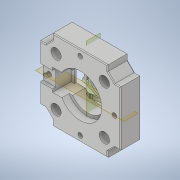
# Autodesk Inventor part: 20_Cube_Insert_VCA_base_upper_v0
Saved by Autodesk Inventor 2022.3 (Build 263350000, 350)
## iProperties
Created: 2019-07-01
Part Number: 20_Cube_Insert_VCA_base_upper_v0
Material: Generic
Document SubType Name: Modeling
Designer: diederichbenedict
Density: 1 g/cm^3
Appearance: Default
Author: diederichbenedict
Autodesk Inventor part; units mm, degrees
ref_plane "YZ Plane" through (0, 0, 0) normal (1, 0, 0) x (0, 1, 0)
ref_plane "XZ Plane" through (0, 0, 0) normal (0, 1, 0) x (-1, 0, 0)
ref_plane "Work Plane1" through (-56.3599, 0, 22) normal (0, 0, -1) x (-1, 0, 0)
sketch "Sketch1" plane through (-56.3599, 0, 22) normal (0, 0, -1) x (-1, 0, 0)
  line L0 (-4.0299, -0.3538) -> (-2.2322, 1.4439) construction
  arc A0 (-1.4439, 2.2322) -> (-2.2322, 1.4439) centre (-0.9299, 0.9299) ccw construction
  line L1 (-1.4439, 2.2322) -> (0.3538, 4.0299) construction
  line L2 (-37.8299, 42.8299) -> (-37.8299, 37.8299) construction
  line L3 (-37.8299, 37.8299) -> (-42.9208, 37.8299) construction
  line L4 (-37.8299, 42.2137) -> (-37.8299, 45.8299) construction
  line L5 (-37.8299, 45.8299) -> (-4.0299, 45.8299) construction
  line L6 (-4.0299, 45.8299) -> (-4.0299, 42.2137) construction
  line L7 (-4.0299, 4.0299) -> (0.3538, 4.0299) projected
  circle A1 centre (-20.9299, 20.9299) radius 17.5 projected
  line L8 (-20.9299, 58.9723) -> (17.1124, 20.9299) construction
  line L9 (17.1124, 20.9299) -> (-20.9299, -17.1124) construction
  line L10 (-20.9299, -17.1124) -> (-58.9723, 20.9299) construction
  line L11 (-58.9723, 20.9299) -> (-20.9299, 58.9723) construction
  line L12 (-20.9299, 58.9723) -> (-20.9299, -17.1124) construction
  line L13 (17.1124, 20.9299) -> (-58.9723, 20.9299) construction
  line L14 (-20.9299, 58.9723) -> (32.8701, 58.9723) construction
  line L15 (-43.4299, 43.4299) -> (1.5701, 43.4299) construction
  line L16 (1.5701, 43.4299) -> (1.5701, -1.5701) construction
  line L17 (1.5701, -1.5701) -> (-43.4299, -1.5701) construction
  line L18 (-43.4299, -1.5701) -> (-43.4299, 43.4299) construction
  line L19 (-43.4299, 43.4299) -> (1.5701, -1.5701) construction
  line L20 (1.5701, 43.4299) -> (-43.4299, -1.5701) construction
  line L21 (-43.4299, 5.3876) -> (-43.4299, 36.4723)
  line L22 (-43.4299, 36.4723) -> (-36.4723, 43.4299)
  line L23 (-36.4723, 43.4299) -> (-5.3876, 43.4299)
  line L24 (-5.3876, 43.4299) -> (1.5701, 36.4723)
  line L25 (1.5701, 36.4723) -> (1.5701, 5.3876)
  line L26 (1.5701, 5.3876) -> (-5.3876, -1.5701)
  line L27 (-5.3876, -1.5701) -> (-36.4723, -1.5701)
  line L28 (-36.4723, -1.5701) -> (-43.4299, 5.3876)
  line L29 (-4.0299, 42.2137) -> (-37.8299, 42.2137) projected
  line L30 (-4.0299, -0.3538) -> (-4.0299, 4.0299) projected
  circle A2 centre (-20.9299, 20.9299) radius 1.5
  line L31 (-10.9299, 10.9299) -> (-30.9299, 10.9299) construction
  line L32 (-30.9299, 10.9299) -> (-30.9299, 30.9299) construction
  line L33 (-30.9299, 30.9299) -> (-10.9299, 30.9299) construction
  line L34 (-10.9299, 30.9299) -> (-10.9299, 10.9299) construction
  line L35 (-10.9299, 10.9299) -> (-30.9299, 30.9299) construction
  line L36 (-30.9299, 10.9299) -> (-10.9299, 30.9299) construction
  circle A3 centre (-30.9299, 30.9299) radius 1.4
  circle A4 centre (-30.9299, 10.9299) radius 1.4
  circle A5 centre (-10.9299, 10.9299) radius 1.4
  line L37 (-45.8299, 37.8299) -> (-42.0723, 37.8299) construction
  line L38 (-42.1723, 37.7299) -> (-45.8299, 37.7299)
  line L39 (-45.8299, 37.7299) -> (-45.8299, 4.1299)
  line L40 (-45.8299, 4.1299) -> (-42.1723, 4.1299)
  line L41 (-42.1723, 4.1299) -> (-42.1723, 37.7299)
  line L42 (-45.8299, 4.0299) -> (-42.0723, 4.0299) construction
  line L43 (-45.8299, 37.8299) -> (-42.0723, 37.8299) projected
  line L44 (-37.7299, 45.8299) -> (-4.1299, 45.8299)
  line L45 (-4.1299, 45.8299) -> (-4.1299, 42.1723)
  line L46 (-4.1299, 42.1723) -> (-37.7299, 42.1723)
  line L47 (-37.7299, 42.1723) -> (-37.7299, 45.8299)
  line L48 (0.4701, 37.8299) -> (0.4701, 4.0299) construction
  line L49 (0.4701, 4.0299) -> (3.9701, 4.0299) construction
  line L50 (3.9701, 37.8299) -> (3.9701, 4.0299) construction
  line L51 (0.4701, 37.8299) -> (3.9701, 37.8299) construction
  line L52 (-45.8299, -3.9701) -> (-4.0299, -3.9701) construction
  line L53 (0.3124, 37.7299) -> (3.9701, 37.7299)
  line L54 (3.9701, 37.7299) -> (3.9701, 4.1299)
  line L55 (3.9701, 4.1299) -> (0.3124, 4.1299)
  line L56 (0.3124, 4.1299) -> (0.3124, 37.7299)
  line L57 (-4.1713, -0.3538) -> (-37.7299, -0.3538)
  line L58 (-37.7299, -0.3538) -> (-37.7299, -3.9701)
  line L59 (-37.7299, -3.9701) -> (-4.1713, -3.9701)
  line L60 (-4.1713, -3.9701) -> (-4.1713, -0.3538)
  point P0 (-37.8299, 4.0299)
  dimension "d18" = 53.8
  dimension "d19" = 45
  dimension "d20" = 53.8
  dimension "d21" = 45
  dimension "d22" = 45
  dimension "d30" = 20
  dimension "d31" = 20
  dimension "d32" = 2.8
  dimension "d33" = 2.8
  dimension "d34" = 2.8
  dimension "d35" = 3
  dimension "d36" = 0.1
  dimension "d37" = 0.1
  dimension "d38" = 0.1
  dimension "d39" = 0.1
  constraints: 86 end point, 21 point on line, 14 parallel, 8 perpendicular, 7 horizontal, 7 midpoint, 4 centre point, 4 coincident, 1 equal length
  measures "d18" distance of L8.start L8.end
  measures "d19" angle of L8 L14
  measures "d20" distance of L8.end L9.end
  measures "d21" distance of L16.end L17.end
  measures "d22" distance of L15.end L16.end
  measures "d30" distance of L32.end L33.end
  measures "d31" distance of L31.end L32.end
  measures "d32" diameter of A3
  measures "d33" diameter of A4
  measures "d34" diameter of A5
  measures "d35" diameter of A2
  measures "d36" distance between parallel lines of L38 L43
  measures "d37" distance between parallel lines of L40 L42
  measures "d38" distance between parallel lines of L45 L6
  measures "d39" distance between parallel lines of L4 L47
extrude "Extrusion1" add sketch "Sketch1" along normal blind 12.5 contours L30 L26 L57 L28 L41 L22 L46 L24 L56 L7 | L7 L26 L30 | L56 L24 L25 L26 | L26 L25 L24 L53 L54 L55 | L60 L59 L58 L57 L28 L27 L26 | L26 L27 L28 L57 | L46 L22 L29 L24 | L24 L29 L45 | L40 L39 L38 L22 L21 L28 | L28 L21 L22 L41 | L29 L22 L23 L24 | L24 L23 L22 L29 L47 L44 L45 | L47 L29 L22 | A1 | A2 | A3 | A4 | A5
sketch "Skizze4" plane through (-56.3599, 0, 9.5) normal (0, 0, -1) x (-1, 0, 0)
  line L0 (-37.7299, 42.1723) -> (-42.1723, 37.7299) projected
  line L1 (-42.1723, 37.7299) -> (-45.8299, 37.7299) projected
  line L2 (-45.8299, 37.7299) -> (-45.8299, 4.1299) construction
  line L3 (-45.8299, 4.1299) -> (-42.1723, 4.1299) projected
  line L4 (-42.1723, 4.1299) -> (-37.6885, -0.3538) projected
  line L5 (-37.6885, -0.3538) -> (-37.7299, -0.3538) projected
  line L6 (-37.7299, -0.3538) -> (-37.7299, -3.9701) projected
  line L7 (-37.7299, -3.9701) -> (-4.1713, -3.9701) construction
  line L8 (-4.1713, -3.9701) -> (-4.1713, -0.3538) projected
  line L9 (-4.1713, -0.3538) -> (0.3124, 4.1299) projected
  line L10 (0.3124, 4.1299) -> (3.9701, 4.1299) projected
  line L11 (3.9701, 4.1299) -> (3.9701, 37.7299) construction
  line L12 (3.9701, 37.7299) -> (0.3124, 37.7299) projected
  line L13 (0.3124, 37.7299) -> (-4.1299, 42.1723) projected
  line L14 (-4.1299, 42.1723) -> (-4.1299, 45.8299) projected
  line L15 (-4.1299, 45.8299) -> (-37.7299, 45.8299) construction
  line L16 (-37.7299, 45.8299) -> (-37.7299, 42.1723) projected
  line L17 (-37.9299, 46.0299) -> (-3.9299, 46.0299) construction
  line L18 (-3.9299, 46.0299) -> (-3.9299, 42.2551)
  line L19 (-3.9299, 42.2551) -> (0.3953, 37.9299)
  line L20 (0.3953, 37.9299) -> (4.1701, 37.9299)
  line L21 (4.1701, 37.9299) -> (4.1701, 3.9299) construction
  line L22 (4.1701, 3.9299) -> (0.3953, 3.9299)
  line L23 (0.3953, 3.9299) -> (-3.9713, -0.4367)
  line L24 (-3.9713, -0.4367) -> (-3.9713, -4.1701)
  line L25 (-3.9713, -4.1701) -> (-37.9299, -4.1701) construction
  line L26 (-37.9299, -4.1701) -> (-37.9299, -0.3953)
  line L27 (-37.9299, -0.3953) -> (-42.2551, 3.9299)
  line L28 (-42.2551, 3.9299) -> (-46.0299, 3.9299)
  line L29 (-46.0299, 3.9299) -> (-46.0299, 37.9299) construction
  line L30 (-46.0299, 37.9299) -> (-42.2551, 37.9299)
  line L31 (-42.2551, 37.9299) -> (-37.9299, 42.2551)
  line L32 (-37.9299, 42.2551) -> (-37.9299, 46.0299)
  line L33 (-45.8299, 37.7299) -> (-45.8299, 37.9299)
  line L34 (-4.1299, 45.8299) -> (-37.7299, 45.8299) projected
  line L35 (-37.7299, 45.8299) -> (-37.9299, 45.8299)
  line L36 (-4.1299, 45.8299) -> (-3.9299, 45.8299)
  line L37 (3.9701, 37.7299) -> (3.9701, 37.9299)
  line L38 (3.9701, 4.1299) -> (3.9701, 37.7299) projected
  line L39 (3.9701, 4.1299) -> (3.9701, 3.9299)
  line L40 (-4.1713, -3.9701) -> (-3.9713, -3.9701)
  line L41 (-37.7299, -3.9701) -> (-37.9299, -3.9701)
  line L42 (-45.8299, 4.1299) -> (-45.8299, 3.9299)
  point P0 (-56.3599, 0)
  dimension "d40" = 0.2
  constraints: 48 end point, 12 point on line, 4 perpendicular, 15 other
  measures "d40" distance between parallel lines of L15 L17
extrude "IM_offset" add sketch "Skizze4" against normal up to surface (12.5 mm away)
ref_plane "Arbeitsebene5" through (-35.4299, 3.9299, 22) normal (-1, 0, 0) x (0, 0, 1)
ref_plane "Arbeitsebene6" through (-18.4299, 20.9299, 22) normal (0, 1, 0) x (-1, 0, 0)
sketch "Skizze31" plane through (-56.3599, 0, 9.5) normal (0, 0, -1) x (-1, 0, 0)
  line L0 (3.9701, 3.9299) -> (3.9701, 37.9299) projected
  line L1 (3.9701, 37.9299) -> (0.3953, 37.9299) projected
  line L2 (0.3953, 37.9299) -> (-3.9299, 42.2551) projected
  line L3 (-3.9299, 42.2551) -> (-3.9299, 45.8299) projected
  line L4 (-3.9299, 45.8299) -> (-37.9299, 45.8299) projected
  line L5 (-37.9299, 45.8299) -> (-37.9299, 42.2551) projected
  line L6 (-37.9299, 42.2551) -> (-42.2551, 37.9299) projected
  line L7 (-42.2551, 37.9299) -> (-45.8299, 37.9299) projected
  line L8 (-45.8299, 37.9299) -> (-45.8299, 3.9299) projected
  line L9 (-42.2551, 3.9299) -> (-45.8299, 3.9299) projected
  line L10 (-37.9299, -0.3953) -> (-42.2551, 3.9299) projected
  line L11 (-37.9299, -3.9701) -> (-37.9299, -0.3953) projected
  line L12 (-3.9713, -3.9701) -> (-37.9299, -3.9701) projected
  line L13 (-3.9713, -3.9701) -> (-3.9713, -0.4367) projected
  line L14 (-3.9713, -0.4367) -> (0.3953, 3.9299) projected
  line L15 (0.3953, 3.9299) -> (3.9701, 3.9299) projected
  circle A0 centre (-20.9506, 20.9092) radius 11.5
  arc A1 (-17.516, 31.8843) -> (-32.4478, 21.1639) centre (-20.9506, 20.9092) ccw projected
  point P0 (-56.3599, 0)
  dimension "d181" = 23
  constraints: 1 centre point
  measures "d181" diameter of A0
extrude "Extrusion26" cut sketch "Skizze31" against normal blind 10 contours A0
chamfer "Fase2" distance 0.5 angle 45 33 edges at (-35.4299, 45.8299, 22) (-18.4299, 44.0425, 22) (-16.2673, 40.0925, 22) (-12.3173, 37.9299, 22) (-10.5299, 20.9299, 22) (-12.3173, 3.9299, 22) (-16.2673, 1.7673, 22) (-18.4299, -2.1827, 22) (-35.4092, -3.9701, 22) (-52.3885, -2.2034, 22) (-54.5718, 1.7466, 22) (-58.5425, 3.9299, 22) (-60.3299, 20.9299, 22) (-58.5425, 37.9299, 22) (-54.5925, 40.0925, 22) (-54.5718, 1.7466, 9.5) (-58.5425, 3.9299, 9.5) (-60.3299, 20.9299, 9.5) (-52.3885, -2.2034, 9.5) (-35.4092, -3.9701, 9.5) (-18.4299, -2.1827, 9.5) (-16.2673, 1.7673, 9.5) (-12.3173, 3.9299, 9.5) (-10.5299, 20.9299, 9.5) (-12.3173, 37.9299, 9.5) (-16.2673, 40.0925, 9.5) (-18.4299, 44.0425, 9.5) (-35.4299, 45.8299, 9.5) (-52.4299, 44.0425, 9.5) (-54.5925, 40.0925, 9.5) (-58.5425, 37.9299, 9.5) (-23.9092, 20.9092, 9.5) (-52.4299, 44.0425, 22)
sketch "Skizze32" plane through (-56.3599, 0, 22) normal (0, 0, 1) x (1, 0, 0)
  line L0 (4.8056, 6.489) -> (64.0062, 6.489) construction
  line L1 (64.0062, 6.489) -> (64.0062, -0.9654) construction
  line L2 (64.0062, -0.9654) -> (4.8056, -0.9654) construction
  line L3 (4.8056, -0.9654) -> (4.8056, 6.489) construction
  point P0 (56.3599, 0)
  constraints: 2 other
extrude "Extrusion27" [suppressed]
sketch "Skizze33" plane through (-56.3599, 0, 22) normal (0, 0, 1) x (1, 0, 0)
  circle A0 centre (20.9506, 20.9092) radius 13 construction
  circle A1 centre (20.9506, 20.9092) radius 13.25
  point P0 (56.3599, 0)
  dimension "d189" = 26.5
  constraints: 1 centre point, 1 coincident
  measures "d189" diameter of A1
extrude "Extrusion28" cut sketch "Skizze33" against normal blind 4.5
sketch "Skizze34" plane through (-56.3599, 0, 22) normal (0, 0, 1) x (1, 0, 0)
  arc A0 (13.1444, 27.1592) -> (13.1444, 14.6592) centre (20.9506, 20.9092) ccw projected
  line L0 (13.1444, 27.1592) -> (6.3506, 27.1592) projected
  line L1 (6.3506, 27.1592) -> (6.3506, 14.6592) projected
  line L2 (6.3506, 14.6592) -> (13.1444, 14.6592) projected
  arc A1 (14.2658, 27.6592) -> (14.2658, 14.1592) centre (20.9506, 20.9092) ccw
  line L3 (14.2658, 27.6592) -> (5.8506, 27.6592)
  line L4 (5.8506, 27.6592) -> (5.8506, 14.1592)
  line L5 (5.8506, 14.1592) -> (14.2658, 14.1592)
  line L6 (5.8506, 27.6592) -> (3.8506, 27.6592)
  line L7 (3.8506, 27.6592) -> (3.8506, 14.1592)
  line L8 (3.8506, 14.1592) -> (5.8506, 14.1592)
  line L9 (5.8506, 14.1592) -> (5.8506, 27.6592)
  point P0 (56.3599, 0)
  point P1 (5.8506, 14.1592)
  dimension "d192" = 0.5
  dimension "d225" = 2
  constraints: 14 end point, 2 parallel, 2 point on circle, 1 centre point, 1 horizontal, 1 perpendicular, 3 other
  measures "d192" distance between parallel lines of L2 L5
  measures "d225" distance of L8.end L7.end
extrude "Extrusion29" cut sketch "Skizze34" against normal through all contours A0 L2 L1 L0 | A1 L5 L4 L3 | L4 L8 L7 L6
sketch "Skizze35" plane through (-56.3599, 0, 9.5) normal (0, 0, -1) x (-1, 0, 0)
  arc A0 (-11.64, 27.6592) -> (-14.9815, 30.7387) centre (-20.9506, 20.9092) ccw projected
  line L0 (-11.64, 27.6592) -> (-5.8506, 27.6592) projected
  line L1 (-5.8506, 27.6592) -> (-5.8506, 14.1592) projected
  line L2 (-5.8506, 14.1592) -> (-11.64, 14.1592) projected
  arc A1 (-13.1632, 12.4472) -> (-11.64, 14.1592) centre (-20.9506, 20.9092) ccw projected
  line L3 (-13.1632, 12.4472) -> (-26.3558, 14.8447) projected
  line L4 (-26.3558, 14.8447) -> (-25.998, 16.8136) projected
  arc A2 (-25.998, 16.8136) -> (-17.1156, 15.6611) centre (-20.9506, 20.9092) ccw projected
  line L5 (-17.1156, 15.6611) -> (-10.4389, 18.0517) projected
  line L6 (-10.4389, 18.0517) -> (-14.9815, 30.7387) projected
  arc A3 (-21.9739, 27.3282) -> (-27.4131, 20.2121) centre (-20.9506, 20.9092) ccw projected
  line L7 (-27.4131, 20.2121) -> (-28.6812, 13.2345) projected
  line L8 (-28.6812, 13.2345) -> (-15.4226, 10.825) projected
  arc A4 (-32.1727, 18.3961) -> (-15.4226, 10.825) centre (-20.9506, 20.9092) ccw projected
  line L9 (-32.1727, 18.3961) -> (-23.5001, 28.6225) projected
  line L10 (-23.5001, 28.6225) -> (-21.9739, 27.3282) projected
  circle A5 centre (-20.9506, 20.9092) radius 5 projected
  circle A6 centre (-12.7006, 35.1986) radius 1.4 projected
  circle A7 centre (-37.4506, 20.9092) radius 1.4 projected
  circle A8 centre (-12.7006, 6.6198) radius 1.4 projected
  line L11 (-17.516, 31.8843) -> (-12.996, 19.2605) projected
  line L12 (-12.996, 19.2605) -> (-14.88, 18.5859) projected
  arc A9 (-14.88, 18.5859) -> (-18.3232, 26.8545) centre (-20.9506, 20.9092) ccw projected
  line L13 (-18.3232, 26.8545) -> (-23.7318, 31.4414) projected
  line L14 (-23.7318, 31.4414) -> (-32.4478, 21.1639) projected
  arc A10 (-17.516, 31.8843) -> (-32.4478, 21.1639) centre (-20.9506, 20.9092) ccw projected
  circle A11 centre (-20.9506, 20.9092) radius 19.3 projected
  point P0 (-56.3599, 0)
extrude "Extrusion30" add sketch "Skizze35" against normal blind 1
sketch "Skizze37" plane through (-56.3599, 0, 10.5) normal (0, 0, 1) x (1, 0, 0)
  line L0 (24.7456, 12.5193) -> (24.388, 14.4871) projected
  line L1 (15.4226, 10.825) -> (28.6812, 13.2345) projected
  line L2 (25.998, 16.8136) -> (26.7134, 12.8769) projected
  line L3 (26.3558, 14.8447) -> (13.1632, 12.4472) projected
  line L4 (17.0328, 13.1504) -> (17.3904, 11.1826) projected
  line L5 (15.4226, 10.825) -> (15.065, 12.7928) projected
  line L6 (26.319, 28.3907) -> (24.7937, 27.0972) projected
  circle A0 centre (20.9506, 20.9092) radius 5 projected
  arc A1 (13.1632, 12.4472) -> (15.4226, 10.825) centre (20.9506, 20.9092) ccw projected
  line L7 (15.4226, 10.825) -> (28.6812, 13.2345) projected
  line L8 (28.6812, 13.2345) -> (27.4131, 20.2121) projected
  arc A2 (27.4131, 20.2121) -> (21.9739, 27.3282) centre (20.9506, 20.9092) ccw projected
  line L9 (21.9739, 27.3282) -> (23.5001, 28.6225) projected
  line L10 (23.5001, 28.6225) -> (32.1727, 18.3961) projected
  arc A3 (32.1727, 18.3961) -> (32.4478, 21.1639) centre (20.9506, 20.9092) ccw projected
  line L11 (32.4478, 21.1639) -> (23.7318, 31.4414) projected
  line L12 (23.7318, 31.4414) -> (18.3232, 26.8545) projected
  arc A4 (18.3232, 26.8545) -> (14.88, 18.5859) centre (20.9506, 20.9092) ccw projected
  line L13 (14.88, 18.5859) -> (12.996, 19.2605) projected
  line L14 (12.996, 19.2605) -> (17.516, 31.8843) projected
  arc A5 (17.516, 31.8843) -> (14.9815, 30.7387) centre (20.9506, 20.9092) ccw projected
  line L15 (14.9815, 30.7387) -> (10.4389, 18.0517) projected
  line L16 (10.4389, 18.0517) -> (17.1156, 15.6611) projected
  arc A6 (17.1156, 15.6611) -> (25.998, 16.8136) centre (20.9506, 20.9092) ccw projected
  line L17 (25.998, 16.8136) -> (26.3558, 14.8447) projected
  line L18 (26.3558, 14.8447) -> (13.1632, 12.4472) projected
  line L19 (29.6289, 21.3957) -> (31.1542, 22.6892) projected
  line L20 (32.4478, 21.1639) -> (30.9225, 19.8703) projected
  line L21 (21.9739, 27.3282) -> (25.0254, 29.9161) projected
  line L22 (11.7873, 21.8176) -> (13.6702, 21.1434) projected
  line L23 (14.88, 18.5859) -> (11.1131, 19.9347) projected
  line L24 (16.1902, 28.1816) -> (14.3073, 28.8558) projected
  line L25 (14.9815, 30.7387) -> (16.8644, 30.0645) projected
  point P0 (56.3599, 0)
  point P1 (24.7937, 27.0972)
  point P2 (26.319, 28.3907)
extrude "Extrusion31" cut sketch "Skizze37" against normal blind 0.5 contours L0 L3 L2 L1 | L1 L5 L3 L4 | L21 L11 L6 L10 | L15 L22 L14 L23 | L19 L11 L20 L10 | L15 L25 L14 L24
sketch "Skizze38" plane through (-56.3599, 0, 9.5) normal (0, 0, -1) x (-1, 0, 0)
  circle A0 centre (-35.9092, 5.9092) radius 3.1599
  circle A1 centre (-35.9092, 35.9092) radius 3.1599
  arc A2 (-32.1727, 18.3961) -> (-15.4226, 10.825) centre (-20.9506, 20.9092) ccw projected
  circle A3 centre (-5.9921, 35.9092) radius 3.1599
  circle A4 centre (-5.9921, 5.9092) radius 3.1599
  point P0 (-56.3599, 0)
  point P1 (-9.7286, 23.4223)
  dimension "d207" = 180
  constraints: 4 centre point, 10 other
extrude "Extrusion32" cut sketch "Skizze38" against normal through all
sketch "Skizze39" plane through (-56.3599, 0, 9.5) normal (0, 0, -1) x (-1, 0, 0)
  line L0 (-32.1727, 18.3961) -> (-23.5001, 28.6225) projected
  line L1 (-23.5001, 28.6225) -> (-21.9739, 27.3282) projected
  arc A0 (-21.9739, 27.3282) -> (-27.4131, 20.2121) centre (-20.9506, 20.9092) ccw projected
  line L2 (-27.4131, 20.2121) -> (-28.6812, 13.2345) projected
  line L3 (-28.6812, 13.2345) -> (-15.4226, 10.825) projected
  arc A1 (-32.1727, 18.3961) -> (-15.4226, 10.825) centre (-20.9506, 20.9092) ccw projected
  circle A2 centre (-20.9506, 20.9092) radius 5 projected
  line L4 (-17.516, 31.8843) -> (-12.996, 19.2605) projected
  line L5 (-12.996, 19.2605) -> (-14.88, 18.5859) projected
  arc A3 (-14.88, 18.5859) -> (-18.3232, 26.8545) centre (-20.9506, 20.9092) ccw projected
  line L6 (-18.3232, 26.8545) -> (-23.7318, 31.4414) projected
  line L7 (-23.7318, 31.4414) -> (-32.4478, 21.1639) projected
  arc A4 (-17.516, 31.8843) -> (-32.4478, 21.1639) centre (-20.9506, 20.9092) ccw projected
  line L8 (-4.4713, -3.4701) -> (-37.4299, -3.4701) projected
  line L9 (-4.4713, -0.2296) -> (-4.4713, -3.4701) projected
  line L10 (0.1882, 4.4299) -> (-4.4713, -0.2296) projected
  line L11 (3.4701, 4.4299) -> (0.1882, 4.4299) projected
  line L12 (3.4701, 37.4299) -> (3.4701, 4.4299) projected
  line L13 (0.1882, 37.4299) -> (3.4701, 37.4299) projected
  line L14 (-4.4299, 42.048) -> (0.1882, 37.4299) projected
  line L15 (-4.4299, 45.3299) -> (-4.4299, 42.048) projected
  line L16 (-37.4299, 45.3299) -> (-4.4299, 45.3299) projected
  line L17 (-37.4299, 42.048) -> (-37.4299, 45.3299) projected
  line L18 (-42.048, 37.4299) -> (-37.4299, 42.048) projected
  line L19 (-45.3299, 37.4299) -> (-42.048, 37.4299) projected
  line L20 (-45.3299, 4.4299) -> (-45.3299, 37.4299) projected
  line L21 (-42.048, 4.4299) -> (-45.3299, 4.4299) projected
  line L22 (-37.4299, -0.1882) -> (-42.048, 4.4299) projected
  line L23 (-37.4299, -3.4701) -> (-37.4299, -0.1882) projected
  arc A5 (-13.1632, 12.4472) -> (-11.64, 14.1592) centre (-20.9506, 20.9092) ccw projected
  line L24 (-13.1632, 12.4472) -> (-26.3558, 14.8447) projected
  line L25 (-26.3558, 14.8447) -> (-25.998, 16.8136) projected
  arc A6 (-25.998, 16.8136) -> (-17.1156, 15.6611) centre (-20.9506, 20.9092) ccw projected
  line L26 (-17.1156, 15.6611) -> (-10.4389, 18.0517) projected
  line L27 (-10.4389, 18.0517) -> (-14.9815, 30.7387) projected
  arc A7 (-11.64, 27.6592) -> (-14.9815, 30.7387) centre (-20.9506, 20.9092) ccw projected
  line L28 (-20.9506, -0.304) -> (0.2626, 20.9092) construction
  line L29 (0.2626, 20.9092) -> (-20.9506, 42.1224) construction
  line L30 (-20.9506, 42.1224) -> (-42.1638, 20.9092) construction
  line L31 (-42.1638, 20.9092) -> (-20.9506, -0.304) construction
  line L32 (-20.9506, -0.304) -> (-20.9506, 42.1224) construction
  line L33 (0.2626, 20.9092) -> (-42.1638, 20.9092) construction
  line L34 (-20.9506, -0.304) -> (9.0494, -0.304) construction
  line L35 (-5.8506, 14.1592) -> (-11.64, 14.1592) projected
  line L36 (-11.64, 27.6592) -> (-5.8506, 27.6592) projected
  line L37 (-5.8506, 27.6592) -> (-5.8506, 14.1592) projected
  point P0 (-56.3599, 0)
  dimension "d209" = 30
  dimension "d210" = 45
  dimension "d211" = 30
  constraints: 14 end point, 2 midpoint, 2 parallel, 1 equal length, 1 horizontal, 1 perpendicular
  measures "d209" distance of L28.start L28.end
  measures "d210" angle of L34 L28
  measures "d211" distance of L29.end L28.end
hole "Bohrung2" at (-35.4092, -0.304, 9.5) at (-14.196, 20.9092, 9.5) at (-35.4092, 42.1224, 9.5) at (-56.6224, 20.9092, 9.5) direction (0, 0, 1) diameter 2.8 end through all counterbore diameter 6.5 counterbore depth 3
sketch "Skizze40" plane through (-56.3599, 0, 22) normal (0, 0, 1) x (1, 0, 0)
  circle A0 centre (-0.304, 20.9092) radius 1.4
  line L0 (-6.3758, 15.9092) -> (5.8506, 15.9092)
  line L1 (5.8506, 15.9092) -> (5.8506, 25.9092)
  line L2 (5.8506, 25.9092) -> (-6.3758, 25.9092)
  line L3 (-6.3758, 25.9092) -> (-6.3758, 15.9092)
  circle A1 centre (-0.2626, 20.9092) radius 1.4 projected
  line L4 (-6.3758, 15.9092) -> (5.8506, 25.9092) construction
  line L5 (5.8506, 15.9092) -> (-6.3758, 25.9092) construction
  point P0 (56.3599, 0)
  point P1 (-0.2833, 19.5094)
  point P2 (-0.2833, 22.3091)
  dimension "d219" = 10
  constraints: 12 end point, 2 midpoint, 2 parallel, 1 centre point, 1 perpendicular, 2 other
  measures "d219" distance of L1.end L0.end
extrude "Extrusion33" cut sketch "Skizze40" against normal blind 2 contours A0 A1 | L3 L2 L1 L0 picked at (-0.7364, 20.9092)
chamfer "Fase4" distance 1 angle 45 11 edges at (-47.2079, 35.9092, 9.5) (-58.7272, 23.3856, 9.5) (-54.146, 18.8045, 9.5) (-47.2079, 5.9092, 9.5) (-38.6382, 0.0653, 9.5) (-32.1803, 0.0653, 9.5) (-17.2908, 5.9092, 9.5) (-16.7403, 18.8871, 9.5) (-12.1739, 23.4535, 9.5) (-17.2908, 35.9092, 9.5) (-35.4092, 38.8724, 9.5)
sketch "Sketch41" plane through (-56.3599, 0, 9.5) normal (0, 0, -1) x (-1, 0, 0)
  circle A0 centre (-20.9172, 20.8636) radius 11.518
  point P0 (-56.3599, 0)
  constraints: 1 centre point
extrude "Extrusion34" [suppressed]
body "Solid1"
